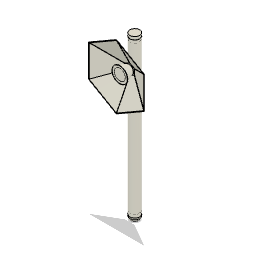
Sarah_Meylan_Objet_Matiere (Autodesk Fusion 360 design; units mm, degrees)
Autodesk Fusion 360 part; units mm, degrees
note: some values were not read from the file. Set by a fixed rule: which face or edge a step refers to.
sketch "Esquisse1" plane through (0, 0, 0) normal (0, 1, 0) x (1, 0, 0)
  circle A0 centre (0, 0) radius 16.5
  dimension "d1" = 33
  constraint coincident A0.centre origin
  measures "d1" diameter of A0
extrude "Extrusion1" add sketch "Esquisse1" along normal blind 520 makes body 1
sketch "Esquisse2" plane through (0, 0, 0) normal (0, 0, 1) x (1, 0, 0)
sketch "Esquisse3" plane through (0, 0, 0) normal (0, 0, 1) x (1, 0, 0)
sketch "Esquisse4" plane through (0, 520, 0) normal (0, 1, 0) x (-1, 0, 0)
  circle A0 centre (0, 0) radius 16.5
  circle A1 centre (0, 0) radius 14.5
  dimension "d5" = 29
  constraint concentric A0 A1
  measures "d5" diameter of A1
extrude "Extrusion2" cut sketch "Esquisse4" against normal blind 575 contours A1 bodies 1
sketch "Esquisse5" plane through (0, 0, 0) normal (0, 0, 1) x (1, 0, 0)
sketch "Esquisse6" plane through (0, 0, 0) normal (0, 1, 0) x (1, 0, 0)
  circle A0 centre (70, 0) radius 16.5
  dimension "d8" = 33
  measures "d8" diameter of A0
extrude "Extrusion3" add sketch "Esquisse6" along normal blind 15 separate body makes body 2
fillet "Congé1" radius 10 1 edges at (54.6166, 0, 5.9667) on bodies 2
sketch "Esquisse7" plane through (0, 15, 0) normal (0, 1, 0) x (-1, 0, 0)
  circle A0 centre (-70, 0) radius 16.5
  circle A1 centre (-70, 0) radius 14.5
  dimension "d13" = 29
  constraint concentric A0 A1
  measures "d13" diameter of A1
extrude "Extrusion4" add sketch "Esquisse7" along normal blind 10 contours A1 bodies 2
move_body "Déplacer1" bodies 2 to x (1, 0, 0) y (0, 1, 0) z (0, 0, 1) at (-70, -15, 0)
sketch "Esquisse8" plane through (0, 0, 0) normal (0, 1, 0) x (1, 0, 0)
  circle A0 centre (66.7253, -0.0835) radius 16.5
  dimension "d16" = 33
  measures "d16" diameter of A0
extrude "Extrusion5" add sketch "Esquisse8" against normal blind 10 separate body makes body 3
sketch "Esquisse9" plane through (0, -10, 0) normal (0, -1, 0) x (1, 0, 0)
  circle A0 centre (66.7253, 0.0835) radius 16.5
  circle A1 centre (66.7253, 0.0835) radius 14.5
  dimension "d19" = 29
  constraint concentric A0 A1
  measures "d19" diameter of A1
extrude "Extrusion6" add sketch "Esquisse9" along normal blind 10 contours A1 bodies 3
move_body "Déplacer2" bodies 3 to x (1, 0, 0) y (0, 1, 0) z (0, 0, 1) at (-66.7518, 530, 0.0095)
sketch "Esquisse10" plane through (0, 0, 0) normal (0, 0, 1) x (1, 0, 0)
sketch "Esquisse11" plane through (0, 10, 0) normal (0, 1, 0) x (-1, 0, 0)
  circle A0 centre (0, 0) radius 14.5
  line L0 (4.6745, -2.0186) -> (-5.3371, -2.0186)
  line L1 (-5.3371, -2.0186) -> (-5.3371, 1.9814)
  line L2 (-5.3371, 1.9814) -> (4.6745, 1.9814)
  line L3 (4.6745, 1.9814) -> (4.6745, -2.0186)
  dimension "d22" = 4
  constraint horizontal L0
  constraint vertical L1
  constraint horizontal L2
  constraint vertical L3
  measures "d22" distance of L0.start L2.end
extrude "Extrusion7" cut sketch "Esquisse11" against normal blind 48 contours L0 L1 L2 L3 bodies 2
sketch "Esquisse12" plane through (0, 10, 0) normal (0, 1, 0) x (-1, 0, 0)
  line L0 (-5.3371, -2.0186) -> (-5.3371, 1.9814)
  line L1 (-5.3371, 1.9814) -> (4.6745, 1.9814)
  line L2 (4.6745, 1.9814) -> (4.6745, -2.0186)
  line L3 (4.6745, -2.0186) -> (-5.3371, -2.0186)
  circle A0 centre (0, 0) radius 14.5
  circle A1 centre (0, 0) radius 12.5
  dimension "d25" = 25
  constraint coincident A0.centre A1.centre
  measures "d25" diameter of A1
extrude "Extrusion8" cut sketch "Esquisse12" against normal blind 22 contours A1 bodies 2
sketch "Esquisse13" plane through (0, 0, 0) normal (0, 0, 1) x (1, 0, 0)
  line L0 (15.6837, 384.765, 17) -> (-0.6149, 393.465, 17)
  line L1 (-0.6149, 393.465, 17) -> (-16.2986, 383.7, 17)
  line L2 (-16.2986, 383.7, 17) -> (-15.6837, 365.235, 17)
  line L3 (-15.6837, 365.235, 17) -> (0.6149, 356.535, 17)
  line L4 (0.6149, 356.535, 17) -> (16.2986, 366.3, 17)
  line L5 (16.2986, 366.3, 17) -> (15.6837, 384.765, 17)
  point P0 (0, 375)
  dimension "d28" = 16
sketch "Esquisse13 (curves 17 mm off its plane)" plane through (0, 0, 17) normal (0, 0, 1) x (1, 0, 0)
  line L0 (15.6837, 384.765) -> (-0.6149, 393.465)
  line L1 (-0.6149, 393.465) -> (-16.2986, 383.7)
  line L2 (-16.2986, 383.7) -> (-15.6837, 365.235)
  line L3 (-15.6837, 365.235) -> (0.6149, 356.535)
  line L4 (0.6149, 356.535) -> (16.2986, 366.3)
  line L5 (16.2986, 366.3) -> (15.6837, 384.765)
extrude "Extrusion9" add sketch "Esquisse13 (curves 17 mm off its plane)" along normal blind 45 draft 60 separate body makes body 4
move_face "DéplacerFace1" to x (0.997564, -0.069756, 0) y (0.069756, 0.997564, 0) z (0, 0, 1) at (-27.9731, 3.4412, 0) 1 faces at (-30.695, 355.8886, 62) on bodies 4
move_face "DéplacerFace2" to x (0.939693, -0.34202, 0) y (0.34202, 0.939693, 0) z (0, 0, 1) at (-165.5554, 27.9187, 0) 1 faces at (-30.695, 355.8886, 62) on bodies 4
move_body "Déplacer3" bodies 4 to x (0.999848, -0.017452, 0) y (0.017452, 0.999848, 0) z (0, 0, 1) at (-4.6671, -1.6295, 0)
move_face "DéplacerFace3" by (0, 50, 0) 1 faces at (-29.1464, 354.7406, 62) on bodies 4
move_body "Déplacer4" bodies 4 to x (1, 0, 0) y (0, 1, 0) z (0, 0, 1) at (0, 60, 0)
move_body "Déplacer5" bodies 4 to x (1, 0, 0) y (0, 1, 0) z (0, 0, 1) at (-4, 0, 0)
shell "Coque1" thickness 1 removed faces 1 at (-33.1464, 414.7406, 62) on bodies 4
move_body "Déplacer6" bodies 4 to x (0.999848, -0.017452, 0) y (0.017452, 0.999848, 0) z (0, 0, 1) at (-5.6842, -1.6419, 0)
sketch "Esquisse14" plane through (0, 0, 0) normal (0, 0, 1) x (1, 0, 0)
  circle A0 through (14.6941, 432.2201, 20) (-7.8059, 445.2105, 20) (-7.8059, 419.2297, 20)
  dimension "d32" = 30
sketch "Esquisse14 (curves 20 mm off its plane)" plane through (0, 0, 20) normal (0, 0, 1) x (1, 0, 0)
  circle A0 centre (-0.3059, 432.2201) radius 15
extrude "Extrusion10" add sketch "Esquisse14 (curves 20 mm off its plane)" along normal blind 30 draft 20 separate body makes body 5
shell "Coque2" thickness 7 removed faces 1 at (-2.9905, 417.8824, 50) on bodies 5
sketch "Esquisse15" plane through (0, 0, 27) normal (0, 0, 1) x (1, 0, 0)
  circle A0 centre (-0.3059, 432.2201) radius 10.0985
sketch "Esquisse16" plane through (0, 0, 27) normal (0, 0, 1) x (1, 0, 0)
  circle A0 centre (-0.1112, 431.9611) radius 5.9346
extrude "Extrusion11" cut sketch "Esquisse16" against normal blind 40 bodies 1 4 5
move_body "Déplacer7" bodies 4 5 to x (1, 0, 0) y (0, 1, 0) z (0, 0, 1) at (0, 0, -0.5)
sketch "Esquisse17" plane through (0, 0, 27) normal (0, 0, 1) x (1, 0, 0)
sketch "Esquisse18" plane through (0, 0, 27) normal (0, 0, 1) x (1, 0, 0)
  circle A0 through (25.966, 432.1701, 23) (-12.9458, 454.6358, 23) (-12.9458, 409.7043, 23)
sketch "Esquisse18 (curves 23 mm off its plane)" plane through (0, 0, 50) normal (0, 0, 1) x (1, 0, 0)
  circle A0 centre (0.0248, 432.1701) radius 25.9412
extrude "Extrusion12" add sketch "Esquisse18 (curves 23 mm off its plane)" along normal blind 1 separate body makes body 6
